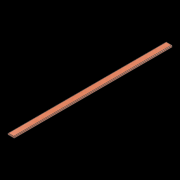
# Autodesk Inventor part: McCrea_doska_walle
Saved by Autodesk Inventor 2021 (Build 250183000, 183)
## iProperties
Created: 2022-01-17
Part Number: McCrea_doska_walle
Material: Generic
Document SubType Name: Modeling
Designer: student
Density: 1 g/cm^3
Appearance: Default
Author: student
Autodesk Inventor part; units mm, degrees
ref_plane "YZ Plane" through (0, 0, 0) normal (1, 0, 0) x (0, 1, 0)
ref_plane "XZ Plane" through (0, 0, 0) normal (0, 1, 0) x (-1, 0, 0)
ref_plane "XY Plane" through (0, 0, 0) normal (0, 0, 1) x (1, 0, 0)
sketch "Sketch1" plane through (0, 0, 0) normal (0, 0, 1) x (1, 0, 0)
  line L0 (-4.125, 0.75) -> (1.875, 0.75)
  line L1 (1.875, 0.75) -> (1.875, -0.75)
  line L2 (1.875, -0.75) -> (-4.125, -0.75)
  line L3 (-4.125, -0.75) -> (-4.125, 0.75)
  point P0 (0, 0)
  dimension "d0" = 6
  dimension "d1" = 1.5
  constraints: 8 end point, 2 parallel, 1 horizontal, 1 perpendicular
  measures "d0" distance of L1.end L2.end
  measures "d1" distance of L0.end L1.end
extrude "Extrusion1" add sketch "Sketch1" along normal blind 150
sketch "Sketch2" plane through (-4.125, -0.75, 0) normal (0, -1, 0) x (1, 0, 0)
  line L0 (0, 0) -> (6, 0) projected
  line L1 (6, 0) -> (6, 150) projected
  line L2 (0, 150) -> (6, 150) projected
  line L3 (0, 0) -> (0, 150) projected
  line L4 (0, 146) -> (6, 146)
  circle A0 centre (3, 148) radius 2
  line L5 (0, 150) -> (6, 150) projected
  point P0 (4.125, 0)
  dimension "d4" = 4
  dimension "d5" = 3
  constraints: 2 end point, 2 tangent, 1 centre point
  measures "d4" distance between parallel lines of L2 L4
  measures "d5" distance from line of L1 A0.centre
fillet "Fillet1" radius 0.5 2 edges at (1.875, 0.75, 75) (-4.125, 0.75, 75)
body "Solid1"
